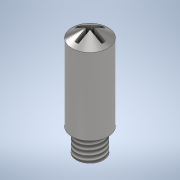
# Autodesk Inventor part: Part32
Saved by Autodesk Inventor 2020 (Build 240168000, 168)
## iProperties
Created: 2021-10-25
Part Number: Part32
Material: Stainless Steel
Document SubType Name: Modeling
Designer: simon.erikssonwestl
Density: 8 g/cm^3
Appearance: Semi-Polished
Author: simon.erikssonwestl
Autodesk Inventor part; units mm, degrees
ref_plane "YZ Plane" through (0, 0, 0) normal (1, 0, 0) x (0, 1, 0)
ref_plane "XZ Plane" through (0, 0, 0) normal (0, 1, 0) x (-1, 0, 0)
ref_plane "XY Plane" through (0, 0, 0) normal (0, 0, 1) x (1, 0, 0)
sketch "Sketch1" plane through (0, 0, 0) normal (0, 1, 0) x (-1, 0, 0)
  circle A0 centre (0, 0) radius 1.5
  dimension "d0" = 3
  constraints: 1 centre point, 1 coincident
  measures "d0" diameter of A0
extrude "Extrusion1" add sketch "Sketch1" along normal blind 2.5
sketch "Sketch2" plane through (0, 2.5, 0) normal (0, 1, 0) x (1, 0, 0)
  circle A0 centre (0, 0) radius 2
  dimension "d3" = 4
  constraints: 1 centre point, 1 coincident
  measures "d3" diameter of A0
extrude "Extrusion2" add sketch "Sketch2" along normal blind 8.5
thread "Thread1" size "M3x0.5" class "6g" standard "ANSI Metric M Profile" length 5.5
sketch "Sketch3" plane through (0, 11, 0) normal (0, 1, 0) x (1, 0, 0)
  circle A0 centre (0, 0) radius 2
  dimension "d8" = 4
  constraints: 1 centre point, 1 coincident
  measures "d8" diameter of A0
extrude "Extrusion3" add sketch "Sketch3" along normal blind 1 draft -60
sketch "Sketch4" plane through (0, 12, 0) normal (0, 1, 0) x (1, 0, 0)
  line L0 (-0.15, 1.5) -> (0.15, 1.5)
  line L1 (0.2, 1.45) -> (0.2, 0.25)
  line L2 (0.15, -1.5) -> (-0.15, -1.5)
  line L3 (-0.2, 0.25) -> (-0.2, 1.45)
  line L4 (-0.2, 1.5) -> (0.2, -1.5) construction
  line L5 (0.2, 1.5) -> (-0.2, -1.5) construction
  line L6 (0.25, 0.2) -> (1.45, 0.2)
  line L7 (1.5, 0.15) -> (1.5, -0.15)
  line L8 (1.45, -0.2) -> (0.25, -0.2)
  line L9 (-1.5, -0.15) -> (-1.5, 0.15)
  circle A0 centre (0, 0) radius 0.2679 projected
  line L10 (-1.5, 0.2) -> (1.5, -0.2) construction
  line L11 (1.5, 0.2) -> (-1.5, -0.2) construction
  arc A1 (-0.15, 1.5) -> (-0.2, 1.45) centre (-0.15, 1.45) ccw
  arc A2 (0.2, 1.45) -> (0.15, 1.5) centre (0.15, 1.45) ccw
  arc A3 (0.2, 0.25) -> (0.25, 0.2) centre (0.25, 0.25) ccw
  arc A4 (1.5, 0.15) -> (1.45, 0.2) centre (1.45, 0.15) ccw
  arc A5 (1.45, -0.2) -> (1.5, -0.15) centre (1.45, -0.15) ccw
  line L12 (0.2, -1.45) -> (0.2, -0.25)
  line L13 (-1.45, 0.2) -> (-0.25, 0.2)
  arc A6 (0.25, -0.2) -> (0.2, -0.25) centre (0.25, -0.25) ccw
  arc A7 (-0.25, 0.2) -> (-0.2, 0.25) centre (-0.25, 0.25) ccw
  line L14 (-1.45, -0.2) -> (-0.25, -0.2)
  line L15 (-0.2, -1.45) -> (-0.2, -0.25)
  arc A8 (-0.2, -0.25) -> (-0.25, -0.2) centre (-0.25, -0.25) ccw
  arc A9 (-1.45, 0.2) -> (-1.5, 0.15) centre (-1.45, 0.15) ccw
  arc A10 (-1.5, -0.15) -> (-1.45, -0.2) centre (-1.45, -0.15) ccw
  arc A11 (-0.2, -1.45) -> (-0.15, -1.5) centre (-0.15, -1.45) ccw
  arc A12 (0.15, -1.5) -> (0.2, -1.45) centre (0.15, -1.45) ccw
  point P0 (0.25, 0.2)
  point P1 (0.3698, -0.2)
  point P2 (-0.2, 0.3871)
  dimension "d11" = 0.4
  dimension "d12" = 3
  dimension "d13" = 3
  dimension "d14" = 0.4
  dimension "d15" = 0.05
  dimension "d16" = 0.05
  dimension "d17" = 0.05
  constraints: 32 end point, 27 point on line, 24 point on circle, 24 tangent, 12 centre point, 9 equal radius, 4 midpoint, 4 parallel, 2 horizontal, 2 perpendicular, 1 vertical
  measures "d11" distance of L4.end L5.end
  measures "d12" distance of L5.start L4.end
  measures "d13" distance of L10.end L11.end
  measures "d14" distance of L11.start L10.end
  measures "d15" radius of A1
  measures "d16" radius of A6
  measures "d17" radius of A8
extrude "Extrusion4" cut sketch "Sketch4" against normal blind 1 contours L0 A2 L1 A3 L6 A4 L7 A5 L8 A6 L12 A12 L2 A11 L15 A8 L14 A10 L9 A9 L13 A7 L3 A1 | A0
body "Solid1"
